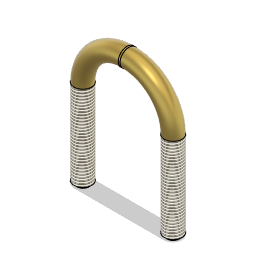
0.880.8262 - Etrier de 10x61x80 - IGTE 21400_17 Rep. 77 (Autodesk Fusion 360 design; units mm, degrees)
Autodesk Fusion 360 part; units mm, degrees
note: some values were not read from the file. Chosen so that the rebuilt part matches the saved one: which face or edge a step refers to; how an offset face is resized.
sketch "Sketch1" plane through (0, 0, 0) normal (0, 0, 1) x (1, 0, 0)
  line L0 (0, 0) -> (60, 0) construction
  line L1 (0, 0) -> (-60, 0) construction
  line L2 (0, 0) -> (0, 60) construction
  line L3 (0, 0) -> (0, -100) construction
  circle A0 centre (0, 19) radius 19 construction
  circle A1 centre (0, 19) radius 24 construction
  line L4 (-25, 0) -> (-25, -30)
  line L5 (25, 0) -> (25, -30)
  line L6 (0, 43) -> (-0.5, 43)
  line L7 (-25, 0) -> (-25, 18.5)
  arc A2 (-0.5, 43) -> (-25, 18.5) centre (-0.5, 18.5) ccw
  line L8 (25, 0) -> (25, 18.5)
  arc A3 (25, 18.5) -> (0.5, 43) centre (0.5, 18.5) ccw
  line L9 (0, 43) -> (0.5, 43)
  line L10 (0, -30) -> (-60, -30) construction
  line L11 (0, -30) -> (60, -30) construction
  dimension "d5" = 38
  dimension "d6" = 5
  dimension "d9" = 24.5
  dimension "d17" = 30
  constraint coincident L0.start L1.start
  constraint horizontal L0
  constraint horizontal L1
  constraint vertical L3
  constraint vertical L2
  constraint coincident L0.start A0
  constraint coincident L2 L6.start
  constraint coincident A1 L6.start
  constraint tangent A1 L6
  constraint perpendicular L2 L6
  constraint perpendicular L6 L7
  constraint tangent L7 A2
  constraint tangent L6 A2
  constraint symmetric L2 L4.start L5.start
  constraint symmetric L2 L6.start L9.start
  constraint symmetric L2 L7.end L8.end
  constraint symmetric L2 L6.end A3.end
  constraint symmetric L2 A2 A3
  constraint parallel L3 L4
  constraint coincident L10 L4.end
  constraint parallel L3 L5
  constraint coincident L11 L5.end
  measures "d5" diameter of A0
  measures "d9" radius of A2
sketch "Sketch2" plane through (0, 0, 0) normal (1, 0, 0) x (0, 0, -1)
  circle A0 centre (0, 43) radius 5
  point P0 (0, 43)
  dimension "d10" = 10
  constraint coincident P0 A0.centre
  measures "d10" diameter of A0
sweep "Sweep1" add profiles "Sketch2" path "Sketch1" along L4 L7 A2 L6 L9 A3 L8 L5 section 1
chamfer "Chamfer1" distance 1.5 angle 45 2 edges at (23.1919, -30, 4.6616) (-26.8081, -30, 4.6616)
thread "Thread1" "ISO Metric profile 10.0 M10x1.5 6g" major diameter 9.85 minor diameter 8.141 pitch 1.5 angle 60 resizes the face on face at (25.2492, -12.8333, -4.9938)
thread "Thread2" "ISO Metric profile 10.0 M10x1.5 6g"
